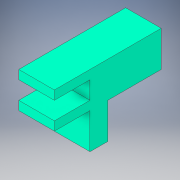
# Autodesk Inventor part: MonsterSupportHolder4
Saved by Autodesk Inventor 2019 (Build 230136000, 136)
## iProperties
Created: 2018-12-06
Part Number: MonsterSupportHolder4
Material: Generic
Document SubType Name: Modeling
Designer: Administrator
Density: 1 g/cm^3
Appearance: Default
Author: Administrator
Autodesk Inventor part; units mm, degrees
ref_plane "YZ Plane" through (0, 0, 0) normal (1, 0, 0) x (0, 1, 0)
ref_plane "XZ Plane" through (0, 0, 0) normal (0, 1, 0) x (-1, 0, 0)
ref_plane "XY Plane" through (0, 0, 0) normal (0, 0, 1) x (1, 0, 0)
sketch "Sketch1" plane through (0, 0, 0) normal (1, 0, 0) x (0, 1, 0)
  line L0 (0, 0) -> (6.35, 0)
  line L1 (6.35, 0) -> (6.35, -6.35)
  line L2 (6.35, -6.35) -> (0, -6.35)
  line L3 (0, -6.35) -> (0, 0)
  dimension "d0" = 6.35
  dimension "d1" = 6.35
  constraints: 8 end point, 2 parallel, 1 horizontal, 1 perpendicular
  measures "d0" distance of L0.start L0.end
  measures "d1" distance of L0.end L1.end
extrude "Extrusion1" add sketch "Sketch1" along normal blind 6.35
sketch "Sketch2" plane through (0, 0, 0) normal (0, 0, 1) x (1, 0, 0)
  line L0 (0, 0) -> (0, 6.35) projected
  line L1 (6.35, 6.35) -> (6.35, 0) projected
  line L2 (0, 4.7625) -> (6.35, 4.7625)
  line L3 (6.35, 4.7625) -> (6.35, 1.5875)
  line L4 (6.35, 1.5875) -> (0, 1.5875)
  line L5 (0, 1.5875) -> (0, 4.7625)
  line L6 (0, 0) -> (6.35, 0) projected
  line L7 (0, 1.5875) -> (0, 0)
  line L8 (0, 0) -> (6.35, 0)
  line L9 (6.35, 0) -> (6.35, 1.5875)
  line L10 (6.35, 4.7625) -> (6.35, 6.35)
  line L11 (0, 6.35) -> (6.35, 6.35) projected
  line L12 (0, 6.35) -> (0, 4.7625)
  line L13 (0, 6.35) -> (6.35, 6.35)
  dimension "d4" = 1.5875
  dimension "d5" = 3.175
  constraints: 20 end point, 4 collinear, 3 perpendicular, 2 parallel, 2 point on line, 1 horizontal
  measures "d4" distance between parallel lines of L6 L4
  measures "d5" distance between parallel lines of L2 L4
extrude "Extrusion2" add sketch "Sketch2" along normal blind 6.35 contours L0 L4 L1 L6 | L0 L11 L1 L2
sketch "Sketch3" plane through (0, 0, -6.35) normal (0, -1, 0) x (1, 0, 0)
  line L0 (6.35, 0) -> (6.35, 12.7) projected
  line L1 (6.35, 6.35) -> (0, 6.35)
  line L2 (0, 6.35) -> (0, 3.175)
  line L3 (0, 3.175) -> (6.35, 3.175)
  line L4 (6.35, 3.175) -> (6.35, 6.35)
  dimension "d8" = 3.175
  dimension "d9" = 6.35
  constraints: 8 end point, 2 parallel, 1 horizontal, 1 midpoint, 1 perpendicular
  measures "d8" distance between parallel lines of L1 L3
  measures "d9" distance between parallel lines of L0 L2
extrude "Extrusion3" add sketch "Sketch3" along normal blind 6.35
sketch "Sketch4" plane through (0, 0, -6.35) normal (0, 0, -1) x (-1, 0, 0)
  line L0 (0, 1.5875) -> (0, 0) projected
  line L1 (-6.35, 4.7625) -> (-6.35, 6.35) projected
  line L2 (0, 0) -> (-6.35, 0)
  line L3 (-6.35, 0) -> (-6.35, 6.35)
  line L4 (-6.35, 6.35) -> (0, 6.35)
  line L5 (0, 6.35) -> (0, 0)
  constraints: 8 end point, 2 parallel, 1 horizontal, 1 perpendicular
extrude "Extrusion4" add sketch "Sketch4" along normal blind 6.35
body "Solid1"
